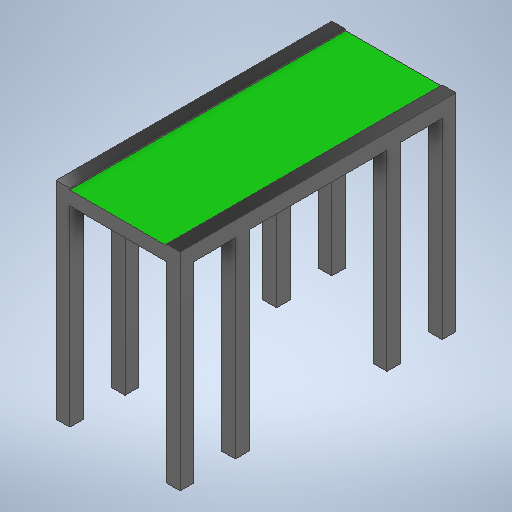
# Autodesk Inventor part: B_Transportadora_Recta_5m
Saved by Autodesk Inventor 2025.2 (Build 292293000, 293)
## iProperties
Created: 2025-01-23
Part Number: B_Transportadora_Recta_5m
Material: Aluminum 6061
Document SubType Name: Modeling
Designer: Proyectos
Density: 2.7 g/cm^3
Appearance: Engine Turned
Author: Proyectos
Autodesk Inventor part; units mm, degrees
ref_plane "YZ Plane" through (0, 0, 0) normal (1, 0, 0) x (0, 1, 0)
ref_plane "XZ Plane" through (0, 0, 0) normal (0, 1, 0) x (-1, 0, 0)
ref_plane "XY Plane" through (0, 0, 0) normal (0, 0, 1) x (1, 0, 0)
sketch "Sketch9" plane through (0, 0, 0) normal (0, 1, 0) x (-1, 0, 0)
  line L0 (0, 0) -> (900, 0)
  line L1 (900, 0) -> (900, -2000)
  line L2 (900, -2000) -> (0, -2000)
  line L3 (0, -2000) -> (0, 0)
  line L4 (900, -2000) -> (800, -2000)
  line L5 (800, -2000) -> (800, 3000)
  line L6 (800, 3000) -> (900, 3000)
  line L7 (900, 3000) -> (900, -2000)
  line L8 (0, -2000) -> (100, -2000)
  line L9 (100, -2000) -> (100, 0)
  line L10 (100, 0) -> (0, 0)
  line L11 (0, 0) -> (0, -2000)
  point P0 (100, -2000)
  point P1 (800, 0)
  dimension "d70" = 900
  dimension "d71" = 100
  dimension "d72" = 100
  dimension "d106" = 2000
  constraints: 24 end point, 6 parallel, 3 horizontal, 3 perpendicular
  measures "d70" distance of L1.end L2.end
  measures "d71" distance of L5.end L6.end
  measures "d72" distance of L10.end L9.end
  measures "d106" distance of L2.end L0.start
extrude "Extrusion6" add sketch "Sketch9" along normal blind 1790 contours L0 L9 L2 L3 | L0 L1 L2 L5
sketch "Sketch10" plane through (0, 0, 0) normal (1, 0, 0) x (0, 0, -1)
  line L0 (0, 0) -> (0, 1790) projected
  line L1 (0, 1790) -> (5000, 1790)
  line L2 (5000, 1790) -> (5000, 1290)
  line L3 (5000, 1290) -> (0, 1290)
  line L4 (0, 1290) -> (0, 1790)
  line L5 (0, 1790) -> (5000, 1790)
  line L6 (5000, 1790) -> (5000, 1390)
  line L7 (5000, 1390) -> (0, 1390)
  line L8 (0, 1390) -> (0, 1790)
  line L9 (0, 1790) -> (5000, 1790)
  line L10 (5000, 1790) -> (5000, 1490)
  line L11 (5000, 1490) -> (0, 1490)
  line L12 (0, 1490) -> (0, 1790)
  line L13 (2000, 0) -> (0, 0) projected
  line L14 (0, 0) -> (500, 0)
  line L15 (500, 0) -> (500, 600)
  line L16 (500, 600) -> (0, 600)
  line L17 (0, 600) -> (0, 0)
  line L18 (2000, 0) -> (1500, 0)
  line L19 (1500, 0) -> (1500, 600)
  line L20 (1500, 600) -> (2000, 600)
  line L21 (2000, 600) -> (2000, 0)
  point P0 (5000, 1490)
  point P1 (0, 1490)
  point P2 (0, 1390)
  dimension "d83" = 500
  dimension "d84" = 500
  dimension "d85" = 600
  dimension "d86" = 600
  constraints: 40 end point, 10 parallel, 5 horizontal, 5 perpendicular
  measures "d83" distance of L15.end L16.end
  measures "d84" distance of L19.end L20.end
  measures "d85" distance of L14.end L15.end
  measures "d86" distance of L18.end L19.end
extrude "Extrusion7" add sketch "Sketch10" against normal blind 900 contours L0 L11 L2 L7
sketch "Sketch13" plane through (0, 1790, 0) normal (0, 1, 0) x (1, 0, 0)
  line L0 (-900, 2000) -> (-900, 0) projected
  line L1 (0, 0) -> (0, 2000) projected
  line L2 (-900, 0) -> (0, 0)
  line L3 (0, 0) -> (0, 2000)
  line L4 (0, 2000) -> (-900, 2000)
  line L5 (-900, 2000) -> (-900, 0)
  point P0 (0, 4500)
  constraints: 8 end point, 2 parallel, 1 horizontal, 1 perpendicular
extrude "Extrusion9" cut sketch "Sketch13" against normal blind 290
sketch "Boceto15" plane through (0, 1490, -2000) normal (0, 1, 0) x (1, 0, 0)
  line L0 (-900, 0) -> (-900, 3000) projected
  line L1 (0, 0) -> (-100, 0) projected
  line L2 (-900, 3000) -> (0, 3000)
  line L3 (0, 3000) -> (0, 0)
  line L4 (0, 0) -> (-900, 0)
  line L5 (-900, 0) -> (-900, 3000)
  point P0 (0, -2000)
  point P1 (-900, 0)
  point P2 (-100, 0)
  constraints: 8 end point, 2 parallel, 1 horizontal, 1 perpendicular
extrude "Extrusión11" cut sketch "Boceto15" against normal blind 1500
sketch "Boceto16" plane through (0, 0, 0) normal (1, 0, 0) x (0, 0, -1)
  line L0 (0, 0) -> (500, 0)
  line L1 (2000, 0) -> (0, 0) projected
  line L2 (2000, 0) -> (1500, 0)
  line L3 (0, 1390) -> (2000, 1390) projected
  line L4 (500, 0) -> (400, 0)
  line L5 (400, 0) -> (400, 1390)
  line L6 (400, 1390) -> (500, 1390)
  line L7 (500, 1390) -> (500, 0)
  line L8 (0, 0) -> (100, 0)
  line L9 (100, 0) -> (100, 1390)
  line L10 (100, 1390) -> (0, 1390)
  line L11 (0, 1390) -> (0, 0)
  line L12 (2000, 0) -> (1900, 0)
  line L13 (1900, 0) -> (1900, 1390)
  line L14 (1900, 1390) -> (2000, 1390)
  line L15 (2000, 1390) -> (2000, 0)
  line L16 (1500, 0) -> (1600, 0)
  line L17 (1600, 0) -> (1600, 1390)
  line L18 (1600, 1390) -> (1500, 1390)
  line L19 (1500, 1390) -> (1500, 0)
  point P0 (1600, 1390)
  point P1 (1900, 1390)
  point P2 (1500, 1390)
  dimension "d110" = 500
  dimension "d111" = 500
  dimension "d112" = 100
  dimension "d113" = 100
  dimension "d114" = 100
  dimension "d115" = 100
  constraints: 36 end point, 8 parallel, 6 point on line, 4 horizontal, 4 perpendicular
  measures "d110" distance of L0.start L0.end
  measures "d111" distance of L1.start L2.end
  measures "d112" distance of L5.end L6.end
  measures "d113" distance of L10.end L9.end
  measures "d114" distance of L13.end L14.end
  measures "d115" distance of L18.end L17.end
extrude "Extrusión12" cut sketch "Boceto16" against normal blind 1500 contours L9 L3 L5 L0 | L7 L3 L19 L1 | L17 L3 L13 L1
body "Solid2"
